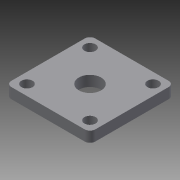
# Autodesk Inventor part: Motor_Shaft_Attachment
Saved by Autodesk Inventor 2015 SP1 (Build 190203100, 203)
## iProperties
Created: 2016-04-10
Part Number: Motor_Shaft_Attachment
Material: Generic
Document SubType Name: Modeling
Designer: guillemd
Density: 1 g/cm^3
Appearance: Default
Author: guillemd
Autodesk Inventor part; units mm, degrees
ref_plane "YZ Plane" through (0, 0, 0) normal (1, 0, 0) x (0, 1, 0)
ref_plane "XZ Plane" through (0, 0, 0) normal (0, 1, 0) x (-1, 0, 0)
ref_plane "XY Plane" through (0, 0, 0) normal (0, 0, 1) x (1, 0, 0)
sketch "Sketch1" plane through (0, 0, 0) normal (0, 1, 0) x (-1, 0, 0)
  line L0 (25.4, 25.4) -> (-25.4, 25.4)
  line L1 (-25.4, 25.4) -> (-25.4, -25.4)
  line L2 (-25.4, -25.4) -> (25.4, -25.4)
  line L3 (25.4, -25.4) -> (25.4, 25.4)
  point P0 (0, 0)
  dimension "d0" = 50.8
  dimension "d1" = 50.8
  dimension "d2" = 25.4
  dimension "d3" = 25.4
  constraints: 8 end point, 2 parallel, 1 horizontal, 1 perpendicular
  measures "d0" distance of L1.end L2.end
  measures "d1" distance of L2.end L0.start
  measures "d2" distance from line of L0 point (0, 0)
  measures "d3" distance from line of L3 point (0, 0)
extrude "Extrusion1" add sketch "Sketch1" along normal blind 6.35
sketch "Sketch2" plane through (0, 6.35, 0) normal (0, 1, 0) x (1, 0, 0)
  point P0 (0, 0)
  point P1 (-19.05, -19.05)
  point P2 (-19.05, 19.05)
  point P3 (19.05, 19.05)
  point P4 (19.05, -19.05)
  dimension "d6" = 38.1
  dimension "d7" = 38.1
  dimension "d8" = 19.05
  dimension "d9" = 19.05
  constraints: 2 horizontal alignment, 2 vertical alignment
  measures "d6" distance of point (-19.05, 19.05) point (-19.05, -19.05)
  measures "d7" distance of point (-19.05, -19.05) point (19.05, -19.05)
  measures "d8" horizontal distance of point (-19.05, -19.05) point (0, 0)
  measures "d9" horizontal distance of point (-19.05, -19.05) point (0, 0)
hole "Hole1" at (-19.05, 6.35, 19.05) at (-19.05, 6.35, -19.05) at (19.05, 6.35, -19.05) at (19.05, 6.35, 19.05) direction (0, -1, 0) diameter 6.7564 end through all clearance for "Flat Head Machine Screw (82)" size "1/4" standard "Ansi Unified Screw Threads"
fillet "Fillet1" radius 3.175 4 edges at (-25.4, 3.175, 25.4) (-25.4, 3.175, -25.4) (25.4, 3.175, -25.4) (25.4, 3.175, 25.4)
sketch "Sketch3" plane through (0, 6.35, 0) normal (0, 1, 0) x (1, 0, 0)
  point P0 (0, 0)
  point P1 (0, 0)
  constraints: 1 coincident
hole "Hole2" at (0, 6.35, 0) direction (0, -1, 0) diameter 13.4874 end through all clearance for "Flat Head Machine Screw (82)" size "1/2" standard "Ansi Unified Screw Threads"
body "Solid1"
